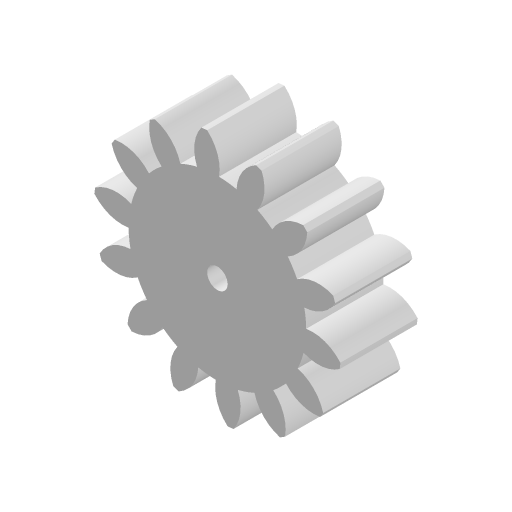
# Autodesk Inventor part: ENGRANE MOTRIZ DE CAJA
Saved by Autodesk Inventor 2024 (Build 280153000, 153)
## iProperties
Created: 2024-06-16
Part Number: ENGRANE MOTRIZ DE CAJA
Material: Generic
Document SubType Name: Modeling
Designer: Jhuliams
Density: 1 g/cm^3
Appearance: Default
Author: Jhuliams
Autodesk Inventor part; units mm, degrees
ref_plane "YZ Plane" through (0, 0, 0) normal (1, 0, 0) x (0, 1, 0)
ref_plane "XZ Plane" through (0, 0, 0) normal (0, 1, 0) x (-1, 0, 0)
ref_plane "XY Plane" through (0, 0, 0) normal (0, 0, 1) x (1, 0, 0)
sketch "Sketch1" plane through (0, 0, 0) normal (0, 0, 1) x (1, 0, 0)
  circle A0 centre (0, 0) radius 17.25
  line L0 (0, 0) -> (42.2346, 0) construction
  line L1 (0, 0) -> (37.3319, 0) construction
  line L2 (0, 0) -> (41.4252, 0) construction
  arc A1 (1.9844, -23.9178) -> (3.1207, -23.7962) centre (0, 0) ccw
  line L3 (0, 0) -> (37.1323, 0) construction
  arc A2 (-0.3152, -17.2471) -> (1.9844, -23.9178) centre (6.7493, -18.5435) ccw
  line L4 (0, 0) -> (32.4854, 0) construction
  arc A3 (3.1207, -23.7962) -> (3.957, -16.79) centre (-2.6733, -19.5516) ccw
  arc A4 (12.1655, -20.6882) -> (13.1365, -20.0856) centre (0, 0) ccw
  arc A5 (7.1993, -15.6759) -> (12.1655, -20.6882) centre (14.1266, -13.7787) ccw
  arc A6 (13.1365, -20.0856) -> (10.8501, -13.4104) centre (6.0746, -18.7753) ccw
  arc A7 (19.937, -13.361) -> (20.5504, -12.3968) centre (0, 0) ccw
  arc A8 (13.2878, -10.9998) -> (19.937, -13.361) centre (18.706, -6.2849) ccw
  arc A9 (20.5504, -12.3968) -> (15.5941, -7.3747) centre (13.6193, -14.2803) ccw
  arc A10 (23.7597, -3.3875) -> (23.894, -2.2527) centre (0, 0) ccw
  arc A11 (16.7446, -4.1451) -> (23.7597, -3.3875) centre (19.5804, 2.4537) ccw
  arc A12 (23.894, -2.2527) -> (17.2496, 0.1217) centre (18.4666, -6.9569) ccw
  arc A13 (22.8766, 7.2569) -> (22.5052, 8.3377) centre (0, 0) ccw
  arc A14 (16.8848, 3.5306) -> (22.8766, 7.2569) centre (16.5767, 10.7064) ccw
  arc A15 (22.5052, 8.3377) -> (15.4885, 7.5939) centre (19.6563, 1.7444) ccw
  arc A16 (17.4624, 16.464) -> (16.6589, 17.2766) centre (0, 0) ccw
  arc A17 (13.6809, 10.507) -> (17.4624, 16.464) centre (10.2898, 16.8385) ccw
  arc A18 (16.6589, 17.2766) -> (10.6598, 13.5621) centre (16.9528, 10.1002) ccw
  arc A19 (8.5896, 22.4102) -> (7.5131, 22.7937) centre (0, 0) ccw
  arc A20 (7.7672, 15.4024) -> (8.5896, 22.4102) centre (1.9648, 19.6355) ccw
  arc A21 (7.5131, 22.7937) -> (3.7198, 16.8442) centre (10.8917, 16.4555) ccw
  arc A22 (-1.9844, 23.9178) -> (-3.1207, 23.7962) centre (0, 0) ccw
  arc A23 (0.3152, 17.2471) -> (-1.9844, 23.9178) centre (-6.7493, 18.5435) ccw
  arc A24 (-3.1207, 23.7962) -> (-3.957, 16.79) centre (2.6733, 19.5516) ccw
  arc A25 (-12.1655, 20.6882) -> (-13.1365, 20.0856) centre (0, 0) ccw
  arc A26 (-7.1993, 15.6759) -> (-12.1655, 20.6882) centre (-14.1266, 13.7787) ccw
  arc A27 (-13.1365, 20.0856) -> (-10.8501, 13.4104) centre (-6.0746, 18.7753) ccw
  arc A28 (-19.937, 13.361) -> (-20.5504, 12.3968) centre (0, 0) ccw
  arc A29 (-13.2878, 10.9998) -> (-19.937, 13.361) centre (-18.706, 6.2849) ccw
  arc A30 (-20.5504, 12.3968) -> (-15.5941, 7.3747) centre (-13.6193, 14.2803) ccw
  arc A31 (-23.7597, 3.3875) -> (-23.894, 2.2527) centre (0, 0) ccw
  arc A32 (-16.7446, 4.1451) -> (-23.7597, 3.3875) centre (-19.5804, -2.4537) ccw
  arc A33 (-23.894, 2.2527) -> (-17.2496, -0.1217) centre (-18.4666, 6.9569) ccw
  arc A34 (-22.8766, -7.2569) -> (-22.5052, -8.3377) centre (0, 0) ccw
  arc A35 (-16.8848, -3.5306) -> (-22.8766, -7.2569) centre (-16.5767, -10.7064) ccw
  arc A36 (-22.5052, -8.3377) -> (-15.4885, -7.5939) centre (-19.6563, -1.7444) ccw
  arc A37 (-17.4624, -16.464) -> (-16.6589, -17.2766) centre (0, 0) ccw
  arc A38 (-13.6809, -10.507) -> (-17.4624, -16.464) centre (-10.2898, -16.8385) ccw
  arc A39 (-16.6589, -17.2766) -> (-10.6598, -13.5621) centre (-16.9528, -10.1002) ccw
  arc A40 (-8.5896, -22.4102) -> (-7.5131, -22.7937) centre (0, 0) ccw
  arc A41 (-7.7672, -15.4024) -> (-8.5896, -22.4102) centre (-1.9648, -19.6355) ccw
  arc A42 (-7.5131, -22.7937) -> (-3.7198, -16.8442) centre (-10.8917, -16.4555) ccw
  point P0 (17.2453, 0.4047)
  point P1 (3.957, -16.79)
  point P2 (15.5941, -7.3747)
  point P3 (-3.957, 16.79)
  point P4 (0.3152, 17.2471)
  point P5 (-7.1993, 15.6759)
  point P6 (-15.4885, -7.5939)
  point P7 (-16.8848, -3.5306)
  point P8 (-10.6598, -13.5621)
  point P9 (17.2496, 0.1217)
  point P10 (15.4885, 7.5939)
  dimension "d2" = 34.5
  dimension "d22" = 48
  dimension "d28" = 360
  constraints: 84 point on circle, 42 centre point, 10 end point, 5 horizontal, 3 coincident, 145 other
  measures "d22" diameter of A1
extrude "Extrusion1" add sketch "Sketch1" along normal blind 15
sketch "Sketch2" plane through (0, 0, 15) normal (0, 0, 1) x (1, 0, 0)
  circle A0 centre (0, 0) radius 2
  dimension "d17" = 4
  constraints: 1 centre point, 1 coincident
  measures "d17" diameter of A0
extrude "Extrusion2" cut sketch "Sketch2" against normal blind 15
body "Solid1"
